Autodesk Fusion 360 part; units mm, degrees
note: some values were not read from the file. Set by a fixed rule: which sketch regions a step uses.
(part 2 of 2)
  constraint coincident L244 L179.end
  constraint coincident L243 L180.end
  constraint tangent L234 A239
  constraint tangent L235 A239
  constraint tangent L235 A240
  constraint tangent L236 A240
  constraint tangent L244 A241
  constraint tangent L243 A241
  constraint tangent L243 A242
  constraint tangent L242 A242
  constraint tangent L233 A243
  constraint tangent L234 A243
  constraint tangent L232 A244
  constraint tangent L233 A244
  constraint tangent L231 A245
  constraint tangent L232 A245
  constraint tangent L230 A246
  constraint tangent L231 A246
  constraint tangent L229 A247
  constraint tangent L230 A247
  constraint tangent L228 A248
  constraint tangent L229 A248
  constraint tangent L228 A249
  constraint tangent L247 A249
  constraint tangent L246 A250
  constraint tangent L247 A250
  constraint tangent L246 A251
  constraint tangent L245 A251
  constraint tangent L244 A252
  constraint tangent L245 A252
  constraint tangent L248 A253
  constraint tangent L242 A253
  constraint tangent L241 A254
  constraint tangent L248 A254
  constraint tangent L249 A255
  constraint tangent L241 A255
  constraint tangent L240 A256
  constraint tangent L249 A256
  constraint tangent L240 A257
  constraint tangent L239 A257
  constraint tangent L239 A258
  constraint tangent L238 A258
  constraint tangent L238 A259
  constraint tangent L237 A259
  constraint tangent L237 A260
  constraint tangent L236 A260
  constraint tangent L250 A261
  constraint tangent L250 A262
  constraint perpendicular L251 L255
  constraint collinear L253 L254
  constraint collinear L255 L256
  constraint tangent L251 A263
  constraint tangent L253 A263
  constraint tangent L251 A264
  constraint tangent L256 A264
  constraint tangent L252 A265
  constraint tangent L254 A265
  constraint tangent L252 A266
  constraint tangent L255 A266
  constraint concentric A3 A267
  constraint concentric A4 A268
  constraint concentric A0 A269
  constraint concentric A1 A270
  constraint concentric A111 A271
  constraint concentric A112 A272
  measures "d1" diameter of A0
  measures "d2" diameter of A1
  measures "d3" diameter of A2
  measures "d4" diameter of A3
  measures "d5" diameter of A4
  measures "d9" diameter of A111
  measures "d12" diameter of A112
  measures "d367" diameter of A267
  measures "d368" diameter of A268
  measures "d369" diameter of A269
  measures "d370" diameter of A270
  measures "d393" diameter of A271
  measures "d394" diameter of A272
extrude "Extrude1" add sketch "mriya" along normal blind 10.5 contours L179 L180 L205 A214 L206 A215 L207 A216 L208 A217 L209 A218 L210 A219 L211 A220 L212 A221 L213 A222 L214 L215 A224 L216 A225 L217 A226 L218 A227 L219 A228 L220 A229 L221 A230 L222 A231 L223 A232 L224 A233 L225 A234 L226 A235 L228 L229 L230 L231 L232 L233 L234 L235 L236 L237 L238 L239 L240 L241 L242 L243 L244 L245 L246 L247 L248 L249 A239 A240 A242 A243 A244 A245 A246 A247 A248 A249 A250 A251 A252 A253 A254 A255 A256 A257 A258 A259 A260 makes body 1
extrude "Extrude2" add sketch "mriya" along normal blind 17 contours L179 L180 L214 A223 L215 L243 L244 A241 bodies 1
extrude "Extrude3" add sketch "mriya" along normal blind 3.7 contours L106 L205 A214 L206 A215 L207 A216 L208 A217 L209 A218 L210 A219 L211 A220 L212 A221 L213 A222 L214 L215 A224 L216 A225 L217 A226 L218 A227 L219 A228 L220 A229 L221 A230 L222 A231 L223 A232 L224 A233 L225 A234 L226 A235 A236 A237 L227 A238 L250 A261 A262 | L106 L214 A223 L215 A236 A237 L227 A238 | L214 L250 A261 A262 | A114 | A115 | A116 | A117 | A271 | A272 bodies 1
extrude "Extrude13" add sketch "mriya" along normal blind 1.8 contours A2 | L109 L110 A118 A119 A120 L187 L188 L191 A198 A199 | A121 L111 A122 L112 A123 L181 L182 L185 A202 A203 | A124 L113 A125 L114 A126 L115 A127 L116 | A128 L117 A129 L118 A130 L119 A131 L120 | A132 L121 A133 A134 L122 L189 L190 L192 A200 A201 | A135 L123 A136 A137 L124 L183 L184 L186 A204 A205 | A138 L125 A139 L126 A140 L127 A141 L128 | A142 L129 A143 L130 A144 L131 A145 L132 | A146 L133 A147 L134 A148 L135 A149 L136 | A150 L137 A151 L138 A152 L139 A153 L140 | A154 L141 A155 L142 A156 L143 A157 L144 | A158 L145 A159 L146 A160 L147 A161 L148 | A162 L149 A163 L150 A164 L151 A165 L152 | A166 L153 A167 L154 A168 L195 L196 L197 A206 A207 | A169 L155 A170 L156 A171 L157 A172 L158 | A173 L159 A174 L160 A175 L201 L202 L203 A210 A211 | A176 L161 A177 L162 A178 L163 A179 L164 | A180 A181 L165 A182 L166 L199 L200 L204 A212 A213 | A183 L167 A184 L168 A185 L169 A186 L170 | A187 A188 L171 A189 L172 L193 L194 L198 A208 A209 | A190 L173 A191 L174 A192 L175 A193 L176 | A194 L177 A195 L251 L253 L256 A263 A264 | A196 L178 A197 L252 L254 L255 A265 A266 bodies 1
extrude "Extrude14" add sketch "mriya" along normal blind 1.7 contours A0 | A1 | A3 | A4 bodies 1
extrude "Extrude6" add sketch "mriya" along normal blind 1 from surface at 14.3 contours L106 L214 A223 L215 A236 A237 L227 A238 bodies 1
extrude "Extrude12" add sketch "mriya" along normal blind 1 from surface at 7.7 contours L214 L250 A261 A262 bodies 1
sketch "power-switch" plane through (-4.4, 0, 0) normal (1, 0, 0) x (0, 1, 0)
  line L0 (19.1932, 0) -> (76.4932, 0)
  line L1 (76.4932, 0) -> (76.4932, 16.8)
  line L2 (76.4932, 16.8) -> (19.1932, 16.8)
  line L3 (19.1932, 16.8) -> (19.1932, 10.5)
  line L4 (36.0932, 5.1) -> (25.6932, 5.1)
  line L5 (25.6932, 5.1) -> (25.6932, 8.1)
  line L6 (25.6932, 8.1) -> (36.0932, 8.1)
  line L7 (36.0932, 8.1) -> (36.0932, 5.1)
  line L8 (37.4932, 3.55) -> (24.2932, 3.55)
  line L9 (23.8932, 3.95) -> (23.8932, 9.25)
  line L10 (24.2932, 9.65) -> (37.4932, 9.65)
  line L11 (37.8932, 9.25) -> (37.8932, 3.95)
  line L12 (19.1932, 10.5) -> (19.1932, 0)
  line L13 (1.9932, 0) -> (76.4932, 0)
  line L14 (76.4932, 0) -> (76.4932, 17)
  line L15 (76.4932, 17) -> (19.2932, 17)
  line L16 (19.2932, 17) -> (19.2932, 10.6)
  line L17 (19.2932, 10.6) -> (1.9932, 10.6)
  line L18 (1.9932, 10.6) -> (1.9932, 0)
  arc A0 (37.8932, 9.25) -> (37.4932, 9.65) centre (37.4932, 9.25) ccw
  arc A1 (37.4932, 3.55) -> (37.8932, 3.95) centre (37.4932, 3.95) ccw
  arc A2 (23.8932, 3.95) -> (24.2932, 3.55) centre (24.2932, 3.95) ccw
  arc A3 (24.2932, 9.65) -> (23.8932, 9.25) centre (24.2932, 9.25) ccw
  line L19 (1.7932, 0) -> (76.6932, 0)
  line L20 (76.6932, 0) -> (76.6932, 17)
  line L21 (76.6932, 17) -> (19.2932, 17)
  line L22 (1.7932, 10.5) -> (1.7932, 0)
  line L23 (19.2932, 17) -> (19.2932, 10.5)
  line L24 (19.2932, 10.5) -> (1.7932, 10.5)
  constraint perpendicular L4 L5
  constraint vertical L5
  constraint perpendicular L5 L6
  constraint vertical L7
  constraint tangent L10 A0
  constraint tangent L11 A0
  constraint tangent L11 A1
  constraint tangent L8 A1
  constraint tangent L8 A2
  constraint tangent L9 A2
  constraint tangent L9 A3
  constraint tangent L10 A3
extrude "Extrude8" cut sketch "power-switch" against normal blind 2.5 contours L4 L5 L6 L7 bodies 1
extrude "Extrude9" cut sketch "power-switch" against normal blind 1 contours L8 L9 L10 L11 A0 A1 A2 A3 bodies 1
chamfer "Chamfer13" distance 0.8 angle 45 4 edges at (-6.9, 25.6932, 6.6) (-6.9, 30.8932, 8.1) (-6.9, 30.8932, 5.1) (-6.9, 36.0932, 6.6) on bodies 1
chamfer "Chamfer14" distance 1 angle 45 8 edges at (-4.4, 30.8932, 3.55) (-4.4, 24.0104, 3.6672) (-4.4, 23.8932, 6.6) (-4.4, 24.0104, 9.5328) (-4.4, 30.8932, 9.65) (-4.4, 37.776, 9.5328) (-4.4, 37.8932, 6.6) (-4.4, 37.776, 3.6672) on bodies 1
sketch "usb-c" plane through (0, 80.6932, 0) normal (0, 1, 0) x (-1, 0, 0)
  line L0 (3.6, 0) -> (36.1295, 0)
  line L1 (3.6, 16.7) -> (3.6, 0)
  line L2 (21.1002, 11) -> (21.1002, 10.2)
  arc A0 (21.1002, 11) -> (19.7003, 12.4) centre (19.7003, 11) ccw
  line L3 (11.7003, 10.2) -> (11.7003, 11)
  line L4 (19.7003, 8.8) -> (13.1003, 8.8)
  line L5 (21.5003, 7.9) -> (11.3002, 7.9)
  arc A1 (11.7003, 10.2) -> (13.1003, 8.8) centre (13.1003, 10.2) ccw
  line L6 (21.9003, 12.9) -> (21.9003, 8.3)
  line L7 (11.3003, 13.3) -> (21.5003, 13.3)
  arc A2 (13.1002, 12.4) -> (11.7002, 11) centre (13.1002, 11) ccw
  arc A3 (19.7003, 8.8) -> (21.1003, 10.2) centre (19.7003, 10.2) ccw
  line L8 (10.9002, 8.3) -> (10.9002, 12.9)
  line L9 (13.1002, 12.4) -> (19.7003, 12.4)
  line L10 (8.6, 0) -> (25.9, 0)
  line L11 (25.9, 10.5) -> (25.9, 16.8)
  line L12 (25.9, 16.8) -> (8.6, 16.8)
  line L13 (8.6, 16.8) -> (8.6, 0)
  line L14 (25.9, 0) -> (25.9, 10.5)
  line L15 (8.6, 0) -> (41.0881, 0)
  line L16 (41.0881, 0) -> (41.0881, 10.5)
  line L17 (41.0881, 10.5) -> (25.9, 10.5)
  line L18 (25.9, 10.5) -> (25.9, 17)
  line L19 (25.9, 17) -> (8.6, 17)
  line L20 (8.6, 17) -> (8.6, 0)
  line L21 (8.6, 0) -> (41.0881, 0)
  line L22 (41.0881, 0) -> (41.0881, 10.6)
  line L23 (41.0881, 10.6) -> (25.8, 10.6)
  line L24 (25.8, 10.6) -> (25.8, 17)
  line L25 (25.8, 17) -> (8.6, 17)
  line L26 (8.6, 17) -> (8.6, 0)
  arc A4 (11.3003, 13.3) -> (10.9002, 12.9) centre (11.3003, 12.9) ccw
  arc A5 (21.9002, 12.9) -> (21.5003, 13.3) centre (21.5003, 12.9) ccw
  arc A6 (10.9002, 8.3) -> (11.3002, 7.9) centre (11.3002, 8.3) ccw
  arc A7 (21.5003, 7.9) -> (21.9002, 8.3) centre (21.5003, 8.3) ccw
  line L27 (8.4, 0) -> (41.0674, 0)
  line L28 (41.0674, 0) -> (41.0674, 10.5)
  line L29 (25.8, 17) -> (8.4, 17)
  line L30 (8.4, 17) -> (8.4, 0)
  line L31 (41.0674, 10.5) -> (25.8, 10.5)
  line L32 (25.8, 10.5) -> (25.8, 17)
  constraint tangent L3 A2
  constraint tangent A2 L9
  constraint tangent A0 L9
  constraint tangent L2 A0
  constraint tangent L4 A3
  constraint tangent L2 A3
  constraint tangent L4 A1
  constraint tangent L3 A1
  constraint perpendicular L6 L7
  constraint perpendicular L5 L8
  constraint horizontal L5
  constraint perpendicular L5 L6
  constraint tangent L7 A4
  constraint tangent L8 A4
  constraint tangent L7 A5
  constraint tangent L6 A5
  constraint tangent L8 A6
  constraint tangent L5 A6
  constraint tangent L5 A7
  constraint tangent L6 A7
extrude "Extrude10" cut sketch "usb-c" against normal blind 2.5 contours L2 A0 L3 L4 A1 A2 A3 L9 bodies 1
extrude "Extrude11" cut sketch "usb-c" against normal blind 1 contours L5 L6 L7 L8 A4 A5 A6 A7 bodies 1
chamfer "Chamfer15" distance 1 angle 45 8 edges at (-16.4002, 80.6932, 7.9) (-11.0174, 80.6932, 8.0172) (-10.9002, 80.6932, 10.6) (-11.0174, 80.6932, 13.1828) (-16.4002, 80.6932, 13.3) (-21.7831, 80.6932, 13.1828) (-21.9003, 80.6932, 10.6) (-21.7831, 80.6932, 8.0172) on bodies 1
chamfer "Chamfer16" distance 0.79 angle 45 3 edges at (-14.85, 78.1932, 14.3) (-6.9, 57.7432, 14.3) (-7.3979, 77.6953, 14.3) on bodies 1
chamfer "Chamfer19" distance 0.8 angle 45 1 edges at (-6.9, 9.5932, 7.7) on bodies 1
chamfer "Chamfer17" distance 1 angle 45 90 edges at (-17.0879, -2.2068, 10.5) (-5.5716, -1.0352, 10.5) (-4.4, 10.5432, 10.5) (-33.4337, 80.6932, 10.5) (-41.4501, 80.7693, 10.5) (-42.3387, 81.5503, 10.5) (-43.8762, 82.7648, 10.5) (-51.4458, 82.9932, 10.5) (-58.2501, 83.0693, 10.5) (-60.2387, 84.9503, 10.5) (-62.8762, 87.2648, 10.5) (-73.4, 87.4932, 10.5) (-83.9238, 87.2648, 10.5) (-86.0613, 85.4503, 10.5) (-87.5499, 84.0693, 10.5) (-94.8542, 83.9932, 10.5) (-102.9238, 83.7648, 10.5) (-107.238, 79.7735, 10.5) (-111.0657, 76.1074, 10.5) (-116.2077, 75.9932, 10.5) (-121.9238, 75.7648, 10.5) (-123.4613, 74.5503, 10.5) (-124.3499, 73.7693, 10.5) (-131.5163, 73.6932, 10.5) (-141.1284, 72.5216, 10.5) (-142.3, 42.8932, 10.5) (-141.1284, 13.2648, 10.5) (-120.4728, 12.0932, 10.5) (-100.9235, 12.4357, 10.5) (-96.4155, 16.4593, 10.5) (-92.7186, 19.941, 10.5) (-84.5898, 20.0932, 10.5) (-75.7143, 19.6842, 10.5) (-70.5474, 11.3702, 10.5) (-65.1972, 2.8703, 10.5) (-56.0828, 2.3932, 10.5) (-48.3499, 2.3171, 10.5) (-47.4613, 1.5361, 10.5) (-45.9238, 0.3216, 10.5) (-37.2542, 0.0932, 10.5) (-29.3499, 0.0171, 10.5) (-28.4613, -0.7639, 10.5) (-26.9238, -1.9784, 10.5) (-17.0879, -2.2068, 0) (-26.9238, -1.9784, 0) (-28.4613, -0.7639, 0) (-29.3499, 0.0171, 0) (-37.2542, 0.0932, 0) (-45.9238, 0.3216, 0) (-47.4613, 1.5361, 0) (-48.3499, 2.3171, 0) (-56.0828, 2.3932, 0) (-65.1972, 2.8703, 0) (-70.5474, 11.3702, 0) (-75.7143, 19.6842, 0) (-84.5898, 20.0932, 0) (-92.7186, 19.941, 0) (-96.4155, 16.4593, 0) (-100.9235, 12.4357, 0) (-120.4728, 12.0932, 0) (-141.1284, 13.2648, 0) (-142.3, 42.8932, 0) (-141.1284, 72.5216, 0) (-131.5163, 73.6932, 0) (-124.3499, 73.7693, 0) (-123.4613, 74.5503, 0) (-121.9238, 75.7648, 0) (-116.2077, 75.9932, 0) (-111.0657, 76.1074, 0) (-107.238, 79.7735, 0) (-102.9238, 83.7648, 0) (-94.8542, 83.9932, 0) (-87.5499, 84.0693, 0) (-86.0613, 85.4503, 0) (-83.9238, 87.2648, 0) (-73.4, 87.4932, 0) (-62.8762, 87.2648, 0) (-60.2387, 84.9503, 0) (-58.2501, 83.0693, 0) (-51.4458, 82.9932, 0) (-43.8762, 82.7648, 0) (-42.3387, 81.5503, 0) (-41.4501, 80.7693, 0) (-24.7337, 80.6932, 0) (-5.5716, 79.5216, 0) (-4.4, 39.2432, 0) (-5.5716, -1.0352, 0) (-4.4, 47.9932, 17) (-5.5716, 79.5216, 17) (-17.1, 80.6932, 17) on bodies 1
fillet "Fillet29" radius 1.2 2 edges at (-4.4, 19.2932, 12.75) (-25.8, 80.6932, 12.75) on bodies 1
chamfer "Chamfer18" distance 1 angle 45 4 edges at (-6.25, 19.2932, 17) (-5.4996, 19.2974, 17) (-25.8, 78.8432, 17) (-25.7958, 79.5936, 17) on bodies 1
chamfer "Chamfer20" distance 0.9 angle 45 6 edges at (-11.1256, 22.891, 0) (-23.6256, 22.891, 0) (-45.9256, 22.941, 0) (-45.9256, 60.941, 0) (-121.9256, 34.941, 0) (-121.9256, 53.941, 0) on bodies 1
sketch "silicone feets" plane through (0, 0, 0) normal (0, 0, -1) x (1, 0, 0)
  circle A0 centre (-120.9, -34.5432) radius 2
  circle A1 centre (-44.9, -22.5432) radius 2
  circle A2 centre (-10.1, -22.4932) radius 2
  line L0 (-8.4, 1.2068) -> (-25.7757, 1.2068)
  arc A3 (-25.7757, 1.2068) -> (-27.1899, 0.621) centre (-25.7757, -0.7932) ccw
  line L1 (-27.1899, 0.621) -> (-28.3184, -0.5074)
  arc A4 (-29.7326, -1.0932) -> (-28.3184, -0.5074) centre (-29.7326, 0.9068) ccw
  line L2 (-29.7326, -1.0932) -> (-44.7757, -1.0932)
  arc A5 (-44.7757, -1.0932) -> (-46.1899, -1.679) centre (-44.7757, -3.0932) ccw
  line L3 (-46.1899, -1.679) -> (-47.3184, -2.8074)
  arc A6 (-48.7326, -3.3932) -> (-47.3184, -2.8074) centre (-48.7326, -1.3932) ccw
  line L4 (-48.7326, -3.3932) -> (-63.4331, -3.3932)
  arc A7 (-63.4331, -3.3932) -> (-65.6097, -4.6635) centre (-63.4331, -5.8932) ccw
  line L5 (-65.6097, -4.6635) -> (-73.7438, -19.0608)
  arc A8 (-77.2264, -21.0932) -> (-73.7438, -19.0608) centre (-77.2264, -17.0932) ccw
  line L6 (-77.2264, -21.0932) -> (-91.9532, -21.0932)
  arc A9 (-94.0745, -20.2145) -> (-91.9532, -21.0932) centre (-91.9532, -18.0932) ccw
  line L7 (-94.0745, -20.2145) -> (-100.1707, -14.1183)
  arc A10 (-100.1707, -14.1183) -> (-102.6456, -13.0932) centre (-102.6456, -16.5932) ccw
  line L8 (-102.6456, -13.0932) -> (-138.3, -13.0932)
  arc A11 (-138.3, -13.0932) -> (-141.3, -16.0932) centre (-138.3, -16.0932) ccw
  line L9 (-141.3, -16.0932) -> (-141.3, -69.6932)
  arc A12 (-141.3, -69.6932) -> (-138.3, -72.6932) centre (-138.3, -69.6932) ccw
  line L10 (-138.3, -72.6932) -> (-124.7326, -72.6932)
  arc A13 (-123.3184, -73.279) -> (-124.7326, -72.6932) centre (-124.7326, -74.6932) ccw
  line L11 (-123.3184, -73.279) -> (-122.1899, -74.4074)
  arc A14 (-122.1899, -74.4074) -> (-120.7757, -74.9932) centre (-120.7757, -72.9932) ccw
  line L12 (-120.7757, -74.9932) -> (-111.6397, -74.9932)
  arc A15 (-109.8719, -75.7254) -> (-111.6397, -74.9932) centre (-111.6397, -77.4932) ccw
  line L13 (-109.8719, -75.7254) -> (-103.19, -82.4074)
  arc A16 (-103.19, -82.4074) -> (-101.7757, -82.9932) centre (-101.7757, -80.9932) ccw
  line L14 (-101.7757, -82.9932) -> (-87.9326, -82.9932)
  arc A17 (-86.5184, -83.579) -> (-87.9326, -82.9932) centre (-87.9326, -84.9932) ccw
  line L15 (-86.5184, -83.579) -> (-84.19, -85.9074)
  arc A18 (-84.19, -85.9074) -> (-82.7757, -86.4932) centre (-82.7757, -84.4932) ccw
  line L16 (-82.7757, -86.4932) -> (-64.0243, -86.4932)
  arc A19 (-64.0243, -86.4932) -> (-62.6101, -85.9074) centre (-64.0243, -84.4932) ccw
  line L17 (-62.6101, -85.9074) -> (-59.2816, -82.579)
  arc A20 (-57.8674, -81.9932) -> (-59.2816, -82.579) centre (-57.8674, -83.9932) ccw
  line L18 (-57.8674, -81.9932) -> (-45.0243, -81.9932)
  arc A21 (-45.0243, -81.9932) -> (-43.6101, -81.4074) centre (-45.0243, -79.9932) ccw
  line L19 (-43.6101, -81.4074) -> (-42.4816, -80.279)
  arc A22 (-41.0674, -79.6932) -> (-42.4816, -80.279) centre (-41.0674, -81.6932) ccw
  line L20 (-41.0674, -79.6932) -> (-8.4, -79.6932)
  arc A23 (-8.4, -79.6932) -> (-5.4, -76.6932) centre (-8.4, -76.6932) ccw
  line L21 (-5.4, -76.6932) -> (-5.4, -1.7932)
  arc A24 (-5.4, -1.7932) -> (-8.4, 1.2068) centre (-8.4, -1.7932) ccw
  circle A25 centre (-22.6, -22.4932) radius 2
  circle A26 centre (-44.9, -60.5432) radius 2
  circle A27 centre (-120.9, -53.5432) radius 2
  circle A28 centre (-10.9, -74.1932) radius 4
  circle A29 centre (-73.4, -80.9932) radius 4
  circle A30 centre (-135.8, -67.1932) radius 4
  circle A31 centre (-135.8, -18.5932) radius 4
  circle A32 centre (-61.6823, -8.8932) radius 4
  circle A33 centre (-10.9, -4.2932) radius 4
  dimension "d374" = 8
  dimension "d375" = 8
  dimension "d376" = 8
  dimension "d377" = 8
  dimension "d378" = 8
  dimension "d379" = 8
  dimension "d380" = 5.5
  dimension "d381" = 5.5
  dimension "d382" = 5.5
  dimension "d383" = 5.5
  dimension "d384" = 5.5
  dimension "d385" = 5.5
  dimension "d386" = 5.5
  dimension "d387" = 5.5
  dimension "d388" = 5.5
  dimension "d389" = 5.5
  dimension "d390" = 5.5
  measures "d374" diameter of A28
  measures "d375" diameter of A29
  measures "d376" diameter of A30
  measures "d377" diameter of A31
  measures "d378" diameter of A32
  measures "d379" diameter of A33
  measures "d380" distance of L20 A28.centre
  measures "d381" distance of L21 A28.centre
  measures "d382" distance of L16 A29.centre
  measures "d383" distance of L10 A30.centre
  measures "d384" distance of L9 A30.centre
  measures "d385" distance of L9 A31.centre
  measures "d386" distance of L8 A31.centre
  measures "d387" distance of L5 A32.centre
  measures "d388" distance of L4 A32.centre
  measures "d389" distance of L0 A33.centre
  measures "d390" distance of L21 A33.centre
extrude "Extrude15" cut sketch "silicone feets" against normal blind 0.8 contours A28 | A29 | A30 | A31 | A32 | A33 bodies 1
extrude "Extrude16" cut sketch "mriya" along normal blind 1 from surface at 2.7 contours A271 | A272 bodies 1
mirror "Mirror1" about plane through (0, 0, 0) normal (1, 0, 0) of bodies 1 makes body 2
named bodies: "Left", "Right"
